pegboard_mount_bracket (Autodesk Fusion 360 design; units mm, degrees)
part number: 2026-09-04-11-03-25-391
Autodesk Fusion 360 part; units mm, degrees
sketch "Plate" plane through (0, 0, 0) normal (0, 1, 0) x (1, 0, 0)
  line L0 (0, 0) -> (7, 0)
  line L1 (7, 0) -> (7, -74)
  line L2 (7, -74) -> (0, -74)
  line L3 (0, -74) -> (0, 0)
  dimension "d58" = 7
  dimension "d59" = 74
  constraint coincident L0.start L3.end
  constraint horizontal L0
  constraint horizontal L2
  constraint vertical L1
  constraint vertical L3
  measures "d58" horizontal distance of L0.start L1.end
  measures "d59" vertical distance of L0.start L1.end
extrude "Plate (1)" add sketch "Plate" along normal mid plane 24
sketch "Hook profile" plane through (0, 0, 0) normal (0, 1, 0) x (1, 0, 0)
  line L0 (0, -72) -> (-8.3, -72)
  line L1 (-8.3, -72) -> (-8.3, -55)
  line L2 (-8.3, -55) -> (-5.3, -55)
  line L3 (-5.3, -55) -> (-3.8, -56.5)
  line L4 (-3.8, -56.5) -> (-3.8, -67)
  line L5 (-3.8, -67) -> (0, -67)
  line L6 (0, -67) -> (0, -72)
  dimension "d62" = 72
  dimension "d63" = 8.3
  dimension "d64" = 3.8
  dimension "d65" = 5
  dimension "d66" = 10.5
  dimension "d67" = 1.5
  dimension "d68" = 1.5
  constraint horizontal L0
  constraint horizontal L2
  constraint horizontal L5
  constraint vertical L1
  constraint vertical L4
  constraint vertical L6
  constraint coincident origin L6
  measures "d62" vertical distance of origin L0.start
  measures "d63" horizontal distance of L0.start L0.end
  measures "d64" horizontal distance of L4.end L5.end
  measures "d65" vertical distance of L0.start L5.end
  measures "d66" vertical distance of L3.end L4.end
  measures "d67" horizontal distance of L2.end L3.end
  measures "d68" vertical distance of L2.end L3.end
extrude "Hook profile (1)" add sketch "Hook profile" along normal mid plane 2.4
pattern_linear "Hook rows" count 2 spacing 25.4 along (0, 0, -1) count 3 spacing 0 along (0, 0, 1) of "Hook profile (1)"
sketch "Nut track 0" plane through (0, 0, 0) normal (0, 1, 0) x (1, 0, 0)
  line L0 (0, -53.545) -> (6, -53.545)
  line L1 (6, -53.545) -> (6, -65.055)
  line L2 (6, -65.055) -> (0, -65.055)
  line L3 (0, -65.055) -> (0, -53.545)
  line L4 (0, -1.75) -> (0, -22.5)
  dimension "d75" = 53.545
  dimension "d76" = 6
  dimension "d77" = 65.055
  constraint horizontal L0
  constraint horizontal L2
  constraint vertical L1
  constraint vertical L3
  constraint collinear L3 L4
  measures "d75" vertical distance of origin L0.start
  measures "d76" horizontal distance of origin L1.end
  measures "d77" vertical distance of origin L1.end
extrude "Nut track 0 (1)" cut sketch "Nut track 0" along normal mid plane 34
sketch "Bolt slot 0" plane through (0, 0, 0) normal (0, 1, 0) x (1, 0, 0)
  line L0 (0, -55.8) -> (8, -55.8)
  line L1 (8, -55.8) -> (8, -62.8)
  line L2 (8, -62.8) -> (0, -62.8)
  line L3 (0, -62.8) -> (0, -55.8)
  line L4 (0, -1.75) -> (0, -22.5)
  dimension "d80" = 55.8
  dimension "d81" = 8
  dimension "d82" = 62.8
  constraint horizontal L0
  constraint horizontal L2
  constraint vertical L1
  constraint vertical L3
  constraint collinear L3 L4
  measures "d80" vertical distance of origin L0.start
  measures "d81" horizontal distance of origin L1.end
  measures "d82" vertical distance of origin L1.end
extrude "Bolt slot 0 (1)" cut sketch "Bolt slot 0" along normal mid plane 14
sketch "Nut track 1" plane through (0, 0, 0) normal (0, 1, 0) x (1, 0, 0)
  line L0 (0, -28.145) -> (6, -28.145)
  line L1 (6, -28.145) -> (6, -39.655)
  line L2 (6, -39.655) -> (0, -39.655)
  line L3 (0, -39.655) -> (0, -28.145)
  line L4 (0, -1.75) -> (0, -22.5)
  dimension "d85" = 28.145
  dimension "d86" = 6
  dimension "d87" = 39.655
  constraint horizontal L0
  constraint horizontal L2
  constraint vertical L1
  constraint vertical L3
  constraint collinear L3 L4
  measures "d85" vertical distance of origin L0.start
  measures "d86" horizontal distance of origin L1.end
  measures "d87" vertical distance of origin L1.end
extrude "Nut track 1 (1)" cut sketch "Nut track 1" along normal mid plane 34
sketch "Bolt slot 1" plane through (0, 0, 0) normal (0, 1, 0) x (1, 0, 0)
  line L0 (0, -30.4) -> (8, -30.4)
  line L1 (8, -30.4) -> (8, -37.4)
  line L2 (8, -37.4) -> (0, -37.4)
  line L3 (0, -37.4) -> (0, -30.4)
  line L4 (0, -1.75) -> (0, -22.5)
  dimension "d90" = 30.4
  dimension "d91" = 8
  dimension "d92" = 37.4
  constraint horizontal L0
  constraint horizontal L2
  constraint vertical L1
  constraint vertical L3
  constraint collinear L3 L4
  measures "d90" vertical distance of origin L0.start
  measures "d91" horizontal distance of origin L1.end
  measures "d92" vertical distance of origin L1.end
extrude "Bolt slot 1 (1)" cut sketch "Bolt slot 1" along normal mid plane 14
equation "bracketWidth = 24.0 mm" comment "bracket width across the upright"
equation "hookTabWidth = slotWidth - 0.8 mm" comment "blade width through the slot"
equation "slotPitchVertical = 25.4 mm" comment "1 inch, measured"
equation "faceMetalThickness = 2.0 mm" comment "upright face metal"
equation "hookThroat = faceMetalThickness + 1.8 mm" comment "gap behind the plate"
equation "hookNeckHeight = 5.0 mm" comment "bears on the slot bottom edge"
equation "hookLipThickness = 4.5 mm" comment "lip thickness behind the face"
equation "hookLipDrop = 12.0 mm" comment "engagement below the neck"
equation "hookLipChamfer = 1.5 mm" comment "lead-in past slot burrs"
equation "topHookNeckTop = 72.0 mm" comment "top row, below the plate top"
equation "hookRows = 2" comment "number of hook rows (pattern count)"
equation "plateThickness = 7.0 mm" comment "the board bolts to this face"
equation "plateHeight = 74.0 mm" comment "plate height, spans the hook rows"
equation "boltSlotHeight = 7.0 mm" comment "1/4-20 clearance, vertical"
equation "boltSlotLength = 14.0 mm" comment "horizontal adjustment range"
equation "nutTrackHeight = 11.51 mm" comment "across flats of a 1/4-20 nut"
equation "nutTrackDepth = 6.0 mm" comment "track depth from the rear face"
equation "slotWidth = 3.2 mm" comment "measured slot width in the upright"
equation "topBoltCentre = 59.3 mm" comment "top bolt, above the plate foot"
equation "d58 = plateThickness"
equation "d59 = plateHeight"
equation "d60 = bracketWidth"
equation "d62 = topHookNeckTop"
equation "d63 = hookThroat + hookLipThickness"
equation "d64 = hookThroat"
equation "d65 = hookNeckHeight"
equation "d66 = hookLipDrop - hookLipChamfer"
equation "d67 = hookLipChamfer"
equation "d68 = hookLipChamfer"
equation "d69 = hookTabWidth"
equation "d71 = hookRows"
equation "d73 = -slotPitchVertical"
equation "d75 = topBoltCentre - nutTrackHeight / 2"
equation "d76 = nutTrackDepth"
equation "d77 = topBoltCentre + nutTrackHeight / 2"
equation "d78 = bracketWidth + 10 mm"
equation "d80 = topBoltCentre - boltSlotHeight / 2"
equation "d81 = plateThickness + 1 mm"
equation "d82 = topBoltCentre + boltSlotHeight / 2"
equation "d83 = boltSlotLength"
equation "d85 = topBoltCentre - 1 * slotPitchVertical - nutTrackHeight / 2"
equation "d86 = nutTrackDepth"
equation "d87 = topBoltCentre - 1 * slotPitchVertical + nutTrackHeight / 2"
equation "d88 = bracketWidth + 10 mm"
equation "d90 = topBoltCentre - 1 * slotPitchVertical - boltSlotHeight / 2"
equation "d91 = plateThickness + 1 mm"
equation "d92 = topBoltCentre - 1 * slotPitchVertical + boltSlotHeight / 2"
equation "d93 = boltSlotLength"
named bodies: "pegboard_mount_bracket"
